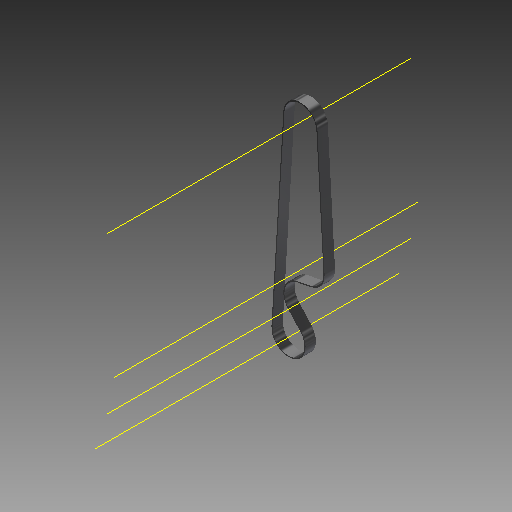
# Autodesk Inventor part: Synchronous Belt
Saved by Autodesk Inventor 2019.4 (Build 234330000, 330)
## iProperties
Created: 2020-01-23
Part Number: Synchronous Belt
Material: Rubber
Document SubType Name: Modeling
Designer: admin
Density: 0.93 g/cm^3
Appearance: Rubber - Black - Version 1.1
Mass: 4.464 g
Surface Area: 105.6 cm^2
Volume: 4.8 cm^3
CustomPartVersion: 1
Author: admin
Autodesk Inventor part; units mm, degrees
sketch "Sketch Path" plane through (0, 0, 0) normal (0, 0, 1) x (1, 0, 0)
  arc A0 (40.1488, -119.2704) -> (67.8239, -109.5642) centre (56.0338, -120.2551) ccw
  arc A1 (83.375, 65.4323) -> (51.6018, 65.4856) centre (67.4868, 64.5009) ccw
  arc A2 (77.4364, -67.2623) -> (90.1848, -50.7282) centre (74.2966, -51.6596) ccw
  arc A3 (64.347, -69.8964) -> (55.6967, -96.19) centre (67.4868, -85.4991) ccw
  line L0 (55.6967, -96.19) -> (67.8239, -109.5642)
  line L1 (40.1488, -119.2704) -> (51.6018, 65.4856)
  line L2 (83.375, 65.4323) -> (90.1848, -50.7282)
  line L3 (77.4364, -67.2623) -> (64.347, -69.8964)
  constraints: 8 end point, 8 point on circle, 4 centre point
ref_plane "Cross Section Plane" through (67.8239, -109.5642, 0) normal (-0.6717, 0.7408, 0) x (0, 0, 1)
ref_plane "Work Plane2" through (56.0338, -120.2551, 0) normal (-1, 0, 0) x (0, 0, 1)
ref_plane "Work Plane3" through (67.4868, 64.5009, 0) normal (-0.3024, -0.9532, 0) x (0, 0, 1)
ref_plane "Work Plane4" through (74.2966, -51.6596, 0) normal (0.2199, 0.9755, 0) x (0, 0, 1)
ref_plane "Work Plane5" through (67.4868, -85.4991, 0) normal (-0.9686, -0.2486, 0) x (0, 0, 1)
sketch "Cross Section" plane through (67.8239, -109.5642, 0) normal (-0.6717, 0.7408, 0) x (0, 0, 1)
  line L0 (-5, 0.5) -> (5, 0.5)
  line L1 (5, 0.5) -> (5, -0.5)
  line L2 (5, -0.5) -> (-5, -0.5)
  line L3 (-5, -0.5) -> (-5, 0.5)
  line L4 (-5, 0) -> (5, 0) construction
  point P0 (0, 0)
  point P1 (0, 0)
  dimension "d0" = 10
  dimension "d4" = 0.5
  dimension "d5" = 0.5
  constraints: 10 end point, 3 midpoint, 2 parallel, 1 coincident, 1 horizontal, 1 perpendicular, 1 other
  measures "d0" distance between parallel lines of L1 L3
  measures "d4" distance between parallel lines of L2 L4
  measures "d5" distance between parallel lines of L4 L0
sweep "Belt" add profiles "Cross Section" path "Sketch Path"
equation "\"d0\" = da_B"
equation "\"d4\" = da_a"
equation "\"d5\" = da_a2"
equation "\"da_B\" = 10"
equation "\"da_pb\" = 5"
equation "\"da_a\" = 0.5"
equation "\"da_S\" = 2.65"
equation "\"da_Beta\" = 20deg"
equation "\"da_Ht\" = 1.2"
equation "\"da_H\" = 3.4"
equation "\"da_a2\" = 0.5"
body "Solid1"
